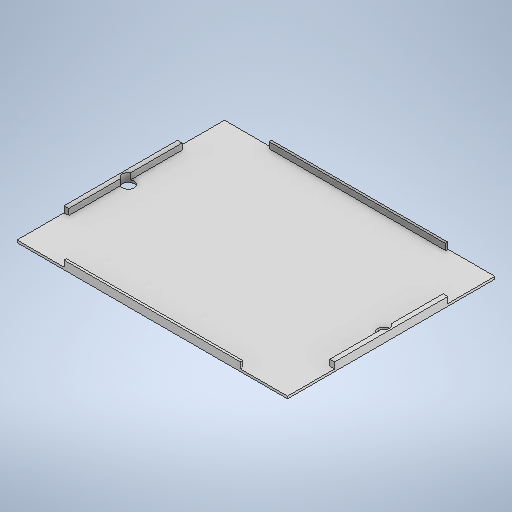
# Autodesk Inventor part: Digital Module Cover V2 - Slim
Saved by Autodesk Inventor 2025 (Build 290162000, 162)
## iProperties
Created: 2025-02-21
Part Number: Digital Module Cover V2 - Slim
Material: Generic
Document SubType Name: Modeling
Designer: Caleb Fangmeier
Density: 1 g/cm^3
Appearance: Default
Author: Caleb Fangmeier
Autodesk Inventor part; units mm, degrees
ref_plane "YZ Plane" through (0, 0, 0) normal (1, 0, 0) x (0, 1, 0)
ref_plane "XZ Plane" through (0, 0, 0) normal (0, 1, 0) x (-1, 0, 0)
ref_plane "XY Plane" through (0, 0, 0) normal (0, 0, 1) x (1, 0, 0)
sketch "Sketch1" plane through (0, 0, 0) normal (0, 1, 0) x (-1, 0, 0)
  line L0 (-28.75, -22.05) -> (28.75, -22.05)
  line L1 (28.75, -22.05) -> (28.75, 22.05)
  line L2 (28.75, 22.05) -> (-28.75, 22.05)
  line L3 (-28.75, 22.05) -> (-28.75, -22.05)
  line L4 (-28.75, -22.05) -> (28.75, 22.05) construction
  line L5 (28.75, -22.05) -> (-28.75, 22.05) construction
  point P0 (0, 0)
  dimension "d2" = 44.1
  dimension "d3" = 57.5
  constraints: 12 end point, 2 midpoint, 2 parallel, 1 horizontal, 1 perpendicular
  measures "d2" distance of L0.end L1.end
  measures "d3" distance of L1.end L2.end
extrude "Extrusion1" add sketch "Sketch1" along normal blind 0.5
sketch "Sketch2" plane through (0, 0.5, 0) normal (0, 1, 0) x (1, 0, 0)
  line L0 (-28.75, 22.05) -> (-28.75, -22.05) projected
  line L1 (28.75, 22.05) -> (-28.75, 22.05) projected
  line L2 (-28.75, -22.05) -> (-27.75, -22.05)
  line L3 (-27.75, -22.05) -> (-27.75, 22.05)
  line L4 (-27.75, 22.05) -> (-28.75, 22.05)
  line L5 (-28.75, 22.05) -> (-28.75, -22.05)
  line L6 (28.75, -22.05) -> (27.75, -22.05)
  line L7 (27.75, -22.05) -> (27.75, 22.05)
  line L8 (27.75, 22.05) -> (28.75, 22.05)
  line L9 (28.75, 22.05) -> (28.75, -22.05)
  point P0 (0, 0)
  dimension "d4" = 1
  dimension "d5" = 1
  constraints: 16 end point, 4 parallel, 3 point on line, 2 horizontal, 2 perpendicular, 1 coincident
  measures "d4" distance between parallel lines of L9 L7
  measures "d5" distance between parallel lines of L0 L3
extrude "Extrusion2" add sketch "Sketch2" along normal blind 1.3
sketch "Sketch3" plane through (0, 0, 0) normal (0, -1, 0) x (1, 0, 0)
  line L0 (28.75, 22.05) -> (28.75, -22.05) projected
  line L1 (-28.75, -22.05) -> (-28.75, 22.05) projected
  point P0 (0, 0)
  point P1 (-27.15, 0)
  point P2 (27.15, 0)
  dimension "d8" = 1.6
  dimension "d9" = 1.6
  constraints: 2 horizontal alignment
  measures "d8" distance from line of point (27.15, 0) L0
  measures "d9" distance from line of point (-27.15, 0) L1
hole "Hole1" at (-27.15, 0, 0) at (27.15, 0, 0) direction (0, 1, 0) diameter 2.5 depth 6.3 tip angle 118
sketch "Sketch4" plane through (0, 0.5, 0) normal (0, 1, 0) x (1, 0, 0)
  line L0 (27.75, -22.05) -> (28.75, -22.05) projected
  line L1 (-27.75, -1.0966) -> (-27.75, -22.05) projected
  line L2 (27.75, -22.05) -> (-27.75, -22.05)
  line L3 (-27.75, -22.05) -> (-27.75, -21.55)
  line L4 (-27.75, -21.55) -> (27.75, -21.55)
  line L5 (27.75, -21.55) -> (27.75, -22.05)
  line L6 (-27.75, 22.05) -> (27.75, 22.05)
  line L7 (27.75, 22.05) -> (27.75, 21.55)
  line L8 (27.75, 21.55) -> (-27.75, 21.55)
  line L9 (-27.75, 21.55) -> (-27.75, 22.05)
  point P0 (0, 0)
  dimension "d17" = 0.5
  dimension "d18" = 0.5
  constraints: 16 end point, 4 parallel, 3 point on line, 2 horizontal, 2 perpendicular, 1 coincident
  measures "d17" distance between parallel lines of L6 L8
  measures "d18" distance between parallel lines of L4 L2
extrude "Extrusion3" add sketch "Sketch4" along normal blind 1.3
sketch "Sketch5" plane through (0, 1.8, 0) normal (0, 1, 0) x (1, 0, 0)
  line L0 (28.75, -22.05) -> (28.75, 22.05) projected
  line L1 (28.75, -22.05) -> (18.75, -22.05)
  line L2 (18.75, -22.05) -> (18.75, -12.05)
  line L3 (18.75, -12.05) -> (28.75, -12.05)
  line L4 (28.75, -12.05) -> (28.75, -22.05)
  line L5 (28.75, 22.05) -> (18.75, 22.05)
  line L6 (18.75, 22.05) -> (18.75, 12.05)
  line L7 (18.75, 12.05) -> (28.75, 12.05)
  line L8 (28.75, 12.05) -> (28.75, 22.05)
  line L9 (-28.75, 22.05) -> (-18.75, 22.05)
  line L10 (-18.75, 22.05) -> (-18.75, 12.05)
  line L11 (-18.75, 12.05) -> (-28.75, 12.05)
  line L12 (-28.75, 12.05) -> (-28.75, 22.05)
  line L13 (-28.75, -22.05) -> (-18.75, -22.05)
  line L14 (-18.75, -22.05) -> (-18.75, -12.05)
  line L15 (-18.75, -12.05) -> (-28.75, -12.05)
  line L16 (-28.75, -12.05) -> (-28.75, -22.05)
  point P0 (0, 0)
  dimension "d21" = 10
  dimension "d22" = 10
  dimension "d23" = 10
  dimension "d24" = 10
  dimension "d25" = 10
  dimension "d26" = 10
  dimension "d27" = 10
  dimension "d28" = 10
  constraints: 32 end point, 8 parallel, 4 horizontal, 4 perpendicular, 2 point on line, 1 coincident
  measures "d21" distance of L1.end L2.end
  measures "d22" distance of L2.end L3.end
  measures "d23" distance of L13.end L14.end
  measures "d24" distance of L9.end L10.end
  measures "d25" distance of L5.end L6.end
  measures "d26" distance of L14.end L15.end
  measures "d27" distance of L10.end L11.end
  measures "d28" distance of L6.end L7.end
extrude "Extrusion4" cut sketch "Sketch5" against normal up to surface (1.3 mm away)
equation "\"d5\" = d4"
equation "\"d18\" = d17"
equation "\"d23\" = d21"
equation "\"d24\" = d21"
equation "\"d25\" = d21"
equation "\"d26\" = d22"
equation "\"d27\" = d22"
equation "\"d28\" = d22"
body "Solid1"
